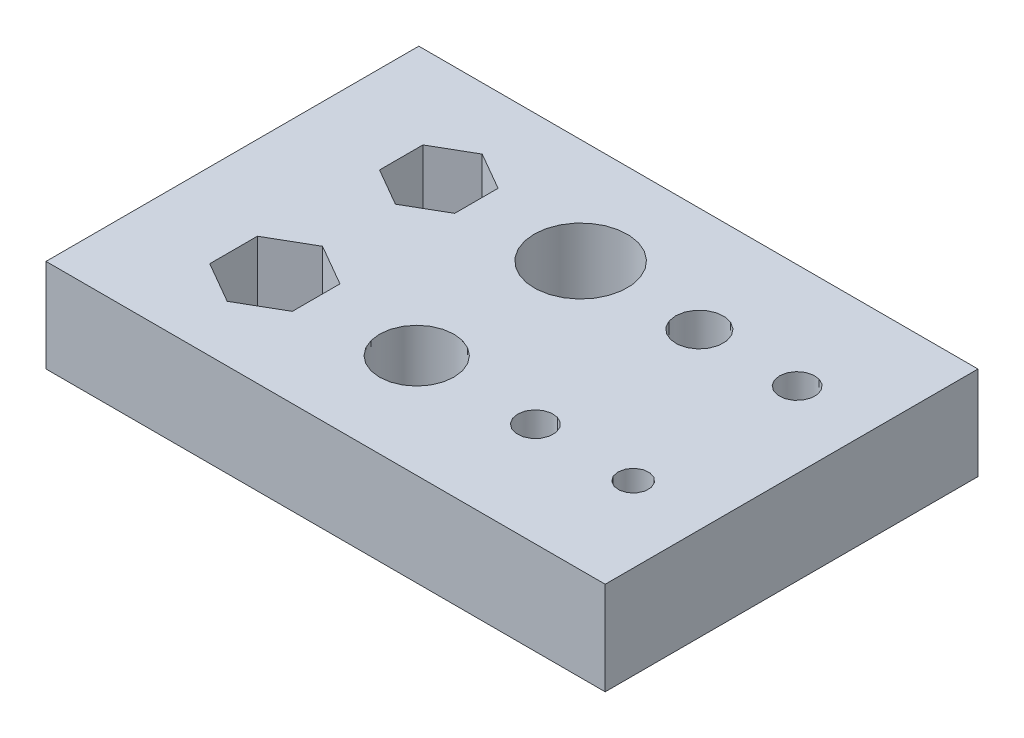
# Autodesk Inventor part: DimensionalCalibration
Saved by Autodesk Inventor 2015 (Build 190159000, 159)
## iProperties
Created: 2015-04-18
Part Number: DimensionalCalibration
Material: Generic
Document SubType Name: Modeling
Designer: doctor
Density: 1 g/cm^3
Appearance: Default
Author: doctor
Autodesk Inventor part; units mm, degrees
ref_plane "YZ Plane" through (0, 0, 0) normal (1, 0, 0) x (0, 1, 0)
ref_plane "XZ Plane" through (0, 0, 0) normal (0, 1, 0) x (-1, 0, 0)
ref_plane "XY Plane" through (0, 0, 0) normal (0, 0, 1) x (1, 0, 0)
sketch "Sketch1" plane through (0, 0, 0) normal (0, 1, 0) x (-1, 0, 0)
  line L0 (0, 0) -> (60, 0)
  line L1 (60, 0) -> (60, -40)
  line L2 (60, -40) -> (0, -40)
  line L3 (0, -40) -> (0, 0)
  line L4 (50.9991, -13.6825) -> (46.57, -16.2397)
  line L5 (46.57, -16.2397) -> (42.1408, -13.6825)
  line L6 (42.1408, -13.6825) -> (42.1408, -8.5682)
  line L7 (42.1408, -8.5682) -> (46.57, -6.011)
  line L8 (46.57, -6.011) -> (50.9991, -8.5682)
  line L9 (50.9991, -8.5682) -> (50.9991, -13.6825)
  line L10 (50.6022, -31.0448) -> (46.57, -33.3728)
  line L11 (46.57, -33.3728) -> (42.5377, -31.0448)
  line L12 (42.5377, -31.0448) -> (42.5377, -26.3887)
  line L13 (42.5377, -26.3887) -> (46.57, -24.0607)
  line L14 (46.57, -24.0607) -> (50.6022, -26.3887)
  line L15 (50.6022, -26.3887) -> (50.6022, -31.0448)
  line L16 (46.57, 0) -> (46.57, -40) construction
  line L17 (60, -11.1253) -> (0, -11.1253) construction
  line L18 (0, -28.7167) -> (60, -28.7167) construction
  line L19 (31.3507, 0) -> (31.3507, -40) construction
  circle A0 centre (31.3507, -11.1253) radius 4
  circle A1 centre (31.3507, -28.7167) radius 5
  line L20 (18.6139, 0) -> (18.6139, -40) construction
  circle A2 centre (18.6139, -11.1253) radius 1.8986
  circle A3 centre (18.6139, -28.7167) radius 2.5527
  line L21 (8.1189, 0) -> (8.1189, -40) construction
  circle A4 centre (8.1189, -11.1253) radius 1.6319
  circle A5 centre (8.1189, -28.7167) radius 1.8987
  point P0 (46.57, -11.1253)
  point P1 (46.57, -28.7167)
  dimension "d0" = 60
  dimension "d1" = 40
  dimension "d2" = 8.8582
  dimension "d3" = 8.0645
  dimension "d4" = 8
  dimension "d5" = 10
  dimension "d6" = 3.7973
  dimension "d7" = 5.1054
  dimension "d8" = 3.2639
  dimension "d9" = 3.7973
  dimension "d23" = 9.3121
  dimension "d24" = 10.2286
  constraints: 44 end point, 28 point on line, 6 centre point, 3 perpendicular, 2 parallel, 1 horizontal, 26 other
  measures "d0" distance of L1.end L2.end
  measures "d1" distance of L0.end L1.end
  measures "d2" distance between parallel lines of L6 L9
  measures "d3" distance between parallel lines of L12 L15
  measures "d4" diameter of A0
  measures "d5" diameter of A1
  measures "d6" diameter of A2
  measures "d7" diameter of A3
  measures "d8" diameter of A4
  measures "d9" diameter of A5
  measures "d23" distance of L11.end L14.end
  measures "d24" distance of L5.end L8.end
extrude "Extrusion1" add sketch "Sketch1" along normal blind 10
body "Solid1"
